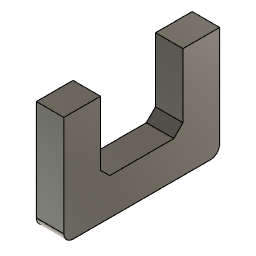
ORIA-tool-set-clip v4 (Autodesk Fusion 360 design; units mm, degrees)
Autodesk Fusion 360 part; units mm, degrees
sketch "Sketch1" plane through (0, 0, 0) normal (0, 0, 1) x (1, 0, 0)
  line L0 (0.75, -2.25) -> (-0.75, -2.25)
  line L1 (-0.75, -2.25) -> (-0.75, 2.25)
  line L2 (-0.75, 2.25) -> (0.75, 2.25)
  line L3 (0.75, 2.25) -> (0.75, -2.25)
  line L4 (0.75, -2.25) -> (-0.75, 2.25) construction
  line L5 (-0.75, -2.25) -> (0.75, 2.25) construction
  line L6 (-0.75, 2.25) -> (0.75, 2.25)
  line L7 (0.75, 2.25) -> (0.75, 4.25)
  line L8 (0.75, 4.25) -> (-0.75, 4.25)
  line L9 (-0.75, 4.25) -> (-0.75, 2.25)
  line L10 (-0.75, -2.25) -> (0.75, -2.25)
  line L11 (0.75, -2.25) -> (0.75, -4.25)
  line L12 (0.75, -4.25) -> (-0.75, -4.25)
  line L13 (-0.75, -4.25) -> (-0.75, -2.25)
  dimension "d1" = 1.5
  dimension "d2" = 4.5
  dimension "d3" = 2
  dimension "d4" = 2
  constraint horizontal L0
  constraint perpendicular L0 L1
  constraint parallel L0 L2
  constraint parallel L1 L3
  constraint coincident L4 origin
  constraint coincident L5 origin
  constraint horizontal L6
  constraint vertical L7
  constraint horizontal L8
  constraint vertical L9
  constraint coincident L2.end L3.start
  constraint horizontal L10
  constraint vertical L11
  constraint horizontal L12
  constraint vertical L13
  constraint coincident L0.start L3.end
  measures "d1" distance of L1.end L2.end
  measures "d2" distance of L0.end L1.end
  measures "d3" distance of L1.end L8.end
  measures "d4" distance of L0.end L12.end
extrude "Extrude1" add sketch "Sketch1" along normal blind 4 contours L0 L10 L11 L12 L13 | L2 L6 L7 L8 L9 makes body 1 at (-0.75, 3.5833, 1.3333) makes body 2 at (0.75, -2.9167, 1.3333)
sketch "Sketch3" plane through (0, 0, 4) normal (0, 0, 1) x (-1, 0, 0)
  line L0 (0.75, -4.25) -> (0.75, -2.25)
  line L1 (0.75, -2.25) -> (-0.75, -2.25)
  line L2 (-0.75, -2.25) -> (-0.75, -4.25)
  line L3 (-0.75, -4.25) -> (0.75, -4.25)
  line L4 (0.75, 4.25) -> (-0.75, 4.25)
  line L5 (-0.75, 4.25) -> (-0.75, 2.25)
  line L6 (0.75, -4.25) -> (0.75, -2.25)
  line L7 (-0.75, -4.25) -> (0.75, -4.25)
  line L8 (0.75, -4.25) -> (-0.75, -4.25)
  line L9 (-0.75, -4.25) -> (-0.75, 4.25)
  line L10 (-0.75, 4.25) -> (0.75, 4.25)
  line L11 (0.75, 4.25) -> (0.75, -4.25)
  constraint horizontal L8
  constraint vertical L9
  constraint horizontal L10
  constraint vertical L11
  constraint coincident L4.end L5.start
  constraint coincident L0.start L3.end
extrude "Extrude2" add sketch "Sketch3" along normal blind 2 bodies 1 2
chamfer "Chamfer1" distance 0.5 angle 45 2 edges at (0, 2.25, 4) (0, -2.25, 4) on bodies 1
fillet "Fillet1" radius 0.5 2 edges at (0, -4.25, 6) (0, 4.25, 6) on bodies 1
move_body "Move1" bodies 1 to x (-1, 0, 0) y (0, 1, 0) z (0, 0, -1) at (0.097, 0, 4.5)
move_body "Align1" bodies 1 to x (1, 0, 0) y (0, 1, 0) z (0, 0, 1) at (0, 0, 1.5)
